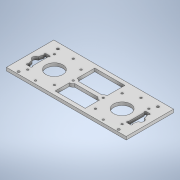
# Autodesk Inventor part: Trunk_lower_waisit_frame
Saved by Autodesk Inventor 2020.4 (Build 244396000, 396)
## iProperties
Created: 2021-09-21
Part Number: Trunk_lower_waisit_frame
Material: アルミニウム 2014-T4
Document SubType Name: Modeling
Designer: Masato Kubotera
Density: 2.8 g/cm^3
Appearance: 滑らか - 淡い灰色
Mass: 76.4309 g
Surface Area: 174.27 cm^2
Volume: 27.2967 cm^3
Description: A2017 T4
Author: Masato Kubotera
Autodesk Inventor part; units mm, degrees
ref_plane "YZ Plane" through (0, 0, 0) normal (1, 0, 0) x (0, 1, 0)
ref_plane "XZ Plane" through (0, 0, 0) normal (0, 1, 0) x (-1, 0, 0)
ref_plane "XY Plane" through (0, 0, 0) normal (0, 0, 1) x (1, 0, 0)
sketch "スケッチ1" plane through (0, 0, 0) normal (0, 0, 1) x (1, 0, 0)
  line L0 (-77.7962, 30.75) -> (77.7962, 30.75)
  line L1 (77.7962, -30.75) -> (-77.7962, -30.75)
  line L2 (-77.7962, 30.75) -> (77.7962, -30.75) construction
  line L3 (77.7962, 30.75) -> (-77.7962, -30.75) construction
  line L4 (0, 30.75) -> (0, -30.75) construction
  circle A0 centre (-44, 2.25) radius 10.5 construction
  line L5 (-57.5, 1.25) -> (-30.5, 1.25) construction
  line L6 (-30.5, 1.25) -> (-30.5, -25.75) construction
  line L7 (-30.5, -25.75) -> (-57.5, -25.75) construction
  line L8 (-57.5, -25.75) -> (-57.5, 1.25) construction
  line L9 (-44, 1.25) -> (-44, -25.75) construction
  line L10 (-57.5, -12.25) -> (-30.5, -12.25) construction
  circle A1 centre (-57.5, 1.25) radius 1.5 construction
  circle A2 centre (-30.5, 1.25) radius 1.5 construction
  line L11 (-67.5, 14.75) -> (-62.5, 14.75) construction
  line L12 (-62.5, 14.75) -> (-62.5, -10.25) construction
  line L13 (-62.5, -10.25) -> (-67.5, -10.25) construction
  line L14 (-67.5, -10.25) -> (-67.5, 14.75) construction
  line L15 (-67.5, 14.75) -> (-62.5, -10.25) construction
  line L16 (-62.5, 14.75) -> (-67.5, -10.25) construction
  line L17 (-67.55, 14.8) -> (-62.45, 14.8)
  line L18 (-62.45, 14.8) -> (-62.45, -10.3)
  line L19 (-62.45, -10.3) -> (-67.55, -10.3)
  line L20 (-67.55, -10.3) -> (-67.55, 14.8)
  line L21 (-67.55, 14.8) -> (-62.45, -10.3) construction
  line L22 (-62.45, 14.8) -> (-67.55, -10.3) construction
  line L23 (-67.55, 2.25) -> (-62.45, 2.25) construction
  line L24 (-65, 14.8) -> (-65, -10.3) construction
  arc A3 (-67.55, 14.8) -> (-67.55, 12.7) centre (-67.55, 13.75) ccw
  arc A4 (-62.45, 12.7) -> (-62.45, 14.8) centre (-62.45, 13.75) ccw
  arc A5 (-67.55, -8.2) -> (-67.55, -10.3) centre (-67.55, -9.25) ccw
  arc A6 (-62.45, -10.3) -> (-62.45, -8.2) centre (-62.45, -9.25) ccw
  circle A7 centre (-65, 27.75) radius 1.55
  line L25 (-10.125, -17.25) -> (-15.125, -17.25) construction
  circle A8 centre (-65, -23.25) radius 1.55
  circle A9 centre (-44, 2.25) radius 11
  line L26 (77.7962, 2.25) -> (-77.7962, 2.25) construction
  line L27 (-60, 14.25) -> (-28, 14.25) construction
  line L28 (-28, 14.25) -> (-28, -28.75) construction
  line L29 (-28, -28.75) -> (-60, -28.75) construction
  line L30 (-60, -28.75) -> (-60, 14.25) construction
  line L31 (-60, 14.25) -> (-28, -28.75) construction
  line L32 (-28, 14.25) -> (-60, -28.75) construction
  line L33 (-77.7962, 30.75) -> (-77.7962, -30.75)
  line L34 (77.7962, 30.75) -> (77.7962, -30.75)
  circle A10 centre (-44, 2.25) radius 12.5 construction
  circle A11 centre (-44, 2.25) radius 20.5 construction
  circle A12 centre (-44, 2.25) radius 28.5 construction
  circle A13 centre (-44, 26.75) radius 1.25
  circle A14 centre (-61.3241, 19.5741) radius 1.25
  circle A15 centre (-68.5, 2.25) radius 1.25
  circle A16 centre (-61.3241, -15.0741) radius 1.25
  circle A17 centre (-44, -22.25) radius 1.25
  circle A18 centre (-26.6759, -15.0741) radius 1.25
  circle A19 centre (-19.5, 2.25) radius 1.25
  circle A20 centre (-26.6759, 19.5741) radius 1.25
  line L35 (-77.7962, -10.0287) -> (-77.7962, -30.75)
  circle A21 centre (57.5, 1.25) radius 1.5 construction
  circle A22 centre (30.5, 1.25) radius 1.5 construction
  line L36 (67.55, 14.8) -> (62.45, 14.8)
  line L37 (62.45, 14.8) -> (62.45, -10.3)
  line L38 (62.45, -10.3) -> (67.55, -10.3)
  line L39 (67.55, -10.3) -> (67.55, 14.8)
  arc A23 (67.55, 12.7) -> (67.55, 14.8) centre (67.55, 13.75) ccw
  arc A24 (62.45, 14.8) -> (62.45, 12.7) centre (62.45, 13.75) ccw
  arc A25 (62.45, -8.2) -> (62.45, -10.3) centre (62.45, -9.25) ccw
  arc A26 (67.55, -10.3) -> (67.55, -8.2) centre (67.55, -9.25) ccw
  circle A27 centre (65, 27.75) radius 1.55
  circle A28 centre (65, -23.25) radius 1.55
  circle A29 centre (44, 2.25) radius 11
  circle A30 centre (44, 26.75) radius 1.25
  circle A31 centre (61.3241, 19.5741) radius 1.25
  circle A32 centre (68.5, 2.25) radius 1.25
  circle A33 centre (61.3241, -15.0741) radius 1.25
  circle A34 centre (44, -22.25) radius 1.25
  circle A35 centre (26.6759, -15.0741) radius 1.25
  circle A36 centre (19.5, 2.25) radius 1.25
  circle A37 centre (26.6759, 19.5741) radius 1.25
  line L40 (77.7962, -10.0287) -> (77.7962, -30.75)
  line L41 (-68.5, 2.25) -> (-73.5, 2.25) construction
  circle A38 centre (-26.6759, -15.0741) radius 6.25 construction
  circle A39 centre (-44, 2.25) radius 24.5 construction
  circle A40 centre (-30.5, -25.75) radius 2.4 construction
  arc A41 (-47.969, 27.2469) -> (-58.8689, 22.732) centre (-44, 2.25) ccw
  arc A42 (-44, 30.75) -> (-47.969, 27.2469) centre (-44, 26.75) ccw
  arc A43 (-58.8689, 22.732) -> (-64.482, 17.1189) centre (-61.3241, 19.5741) ccw
  arc A44 (-64.482, 17.1189) -> (-68.9969, 6.219) centre (-44, 2.25) ccw
  arc A45 (-68.9969, 6.219) -> (-68.9969, -1.719) centre (-68.5, 2.25) ccw
  arc A46 (-68.9969, -1.719) -> (-66.275, -9.7675) centre (-44, 2.25) ccw
  line L42 (-77.7962, -16.309) -> (-77.7962, -10.0287)
  arc A47 (58.8689, 22.732) -> (47.969, 27.2469) centre (44, 2.25) ccw
  arc A48 (47.969, 27.2469) -> (44, 30.75) centre (44, 26.75) ccw
  arc A49 (64.482, 17.1189) -> (58.8689, 22.732) centre (61.3241, 19.5741) ccw
  arc A50 (68.9969, 6.219) -> (64.482, 17.1189) centre (44, 2.25) ccw
  arc A51 (68.9969, -1.719) -> (68.9969, 6.219) centre (68.5, 2.25) ccw
  arc A52 (66.275, -9.7675) -> (68.9969, -1.719) centre (44, 2.25) ccw
  line L43 (77.7962, -16.309) -> (77.7962, -10.0287)
  line L44 (19.5, 25.75) -> (-19.5, 25.75)
  line L45 (-19.5, 25.75) -> (-19.5, 7.25)
  circle A53 centre (-65, 27.75) radius 2.75 construction
  line L46 (-15.1699, 4.75) -> (15.1699, 4.75)
  arc A54 (-15.1699, 4.75) -> (-19.5, 7.25) centre (-19.5, 2.25) ccw
  line L47 (19.5, 25.75) -> (19.5, 7.25)
  arc A55 (19.5, 7.25) -> (15.1699, 4.75) centre (19.5, 2.25) ccw
  line L48 (-15.1699, -0.25) -> (15.1699, -0.25)
  arc A56 (-19.5, -2.75) -> (-15.1699, -0.25) centre (-19.5, 2.25) ccw
  arc A57 (15.1699, -0.25) -> (19.5, -2.75) centre (19.5, 2.25) ccw
  line L49 (-19.5, -2.75) -> (-19.5, -25.75)
  line L50 (-19.5, -25.75) -> (19.5, -25.75)
  line L51 (19.5, -25.75) -> (19.5, -2.75)
  point P0 (0, 0)
  point P1 (-65, 2.25)
  point P2 (-62.45, 12.7)
  point P3 (-62.45, -8.2)
  point P4 (-67.55, -8.2)
  point P5 (-44, -7.25)
  point P6 (62.45, -8.2)
  point P7 (62.45, 12.7)
  point P8 (27.9147, 19.7411)
  point P9 (27.51, 18.6431)
  point P10 (-27.51, 18.6431)
  point P11 (-27.9147, 19.7411)
  point P12 (-26.4271, 21.76)
  point P13 (-26.9247, 21.76)
  point P14 (-27.51, 20.5051)
  point P15 (27.51, 20.5051)
  point P16 (26.9247, 21.76)
  point P17 (26.4271, 21.76)
  point P18 (-47, 30.75)
  point P19 (47, 30.75)
  point P20 (-65, 2.25)
  point P21 (-67.0074, 12.7979)
  point P22 (-67.45, 11.7733)
  point P23 (-67.45, 2.9282)
  point P24 (-67.45, 1.5718)
  point P25 (-67.45, -7.2733)
  point P26 (-67.0074, -8.2979)
  point P27 (67.0074, -8.2979)
  point P28 (67.45, -7.2733)
  point P29 (67.45, 1.5718)
  point P30 (67.45, 2.9282)
  point P31 (67.45, 11.7733)
  point P32 (67.0074, 12.7979)
  point P33 (-67.55, 11.5233)
  point P34 (-65.9794, 14.8)
  point P35 (-67.55, 3.0624)
  point P36 (-67.55, 1.4376)
  point P37 (-67.55, -7.0233)
  point P38 (65.9794, 14.8)
  point P39 (67.55, 11.5233)
  point P40 (67.55, 1.4376)
  point P41 (67.55, 3.0624)
  point P42 (67.55, -7.0233)
  dimension "d3" = 21
  dimension "d4" = 27
  dimension "d5" = 3
  dimension "d7" = 27
  dimension "d8" = 5
  dimension "d9" = 25
  dimension "d10" = 0.05
  dimension "d11" = 0.05
  dimension "d12" = 1.05
  dimension "d13" = 3.1
  dimension "d19" = 3.1
  dimension "d21" = 6
  dimension "d24" = 3
  dimension "d29" = 0.5
  dimension "d34" = 11.5
  dimension "d45" = 32
  dimension "d46" = 43
  dimension "d47" = 9.5
  dimension "d71" = 44
  dimension "d73" = 1
  dimension "d78" = 28.5
  dimension "d79" = 33
  dimension "d80" = 25
  dimension "d81" = 41
  dimension "d82" = 8
  dimension "d84" = 2.5
  dimension "d85" = 24.5
  dimension "d88" = 360
  dimension "d90" = 2
  dimension "d93" = 4
  dimension "d94" = 5
  dimension "d97" = 5
  dimension "d101" = 4.8
  dimension "d105" = 4
  dimension "d106" = 25.31
  dimension "d107" = 4
  dimension "d108" = 25.31
  dimension "d109" = 25.31
  dimension "d110" = 4
  dimension "d113" = 5.5
  dimension "d114" = 5
  dimension "d117" = 5
  dimension "d118" = 5
  dimension "d122" = 5
  dimension "d123" = 16
  dimension "d124" = 13
  dimension "d125" = 67.5
  constraints: 104 end point, 58 centre point, 56 symmetric about line, 50 point on circle, 19 midpoint, 17 coincident, 16 point on line, 10 parallel, 9 perpendicular, 8 horizontal, 4 vertical, 47 other
  measures "d3" diameter of A0
  measures "d4" distance of L6.end L7.end
  measures "d5" diameter of A1
  measures "d7" distance of L6.end L5.end
  measures "d8" distance of L12.end L13.end
  measures "d9" distance of L11.end L12.end
  measures "d10" distance between parallel lines of L17 L11
  measures "d11" distance between parallel lines of L18 L12
  measures "d12" radius of A3
  measures "d13" diameter of A7
  measures "d19" diameter of A8
  measures "d21" vertical distance of L25.start A8.centre
  measures "d24" vertical distance of L4.start A7.centre
  measures "d29" radial gap between concentric circles of A0 A9
  measures "d34" distance from line of A2.centre L13
  measures "d45" distance of L28.end L29.end
  measures "d46" distance of L27.end L28.end
  measures "d47" distance of point (-44, -7.25) A9.centre
  measures "d71" horizontal distance of point (0, 0) A0.centre
  measures "d73" distance of L9.start A9.centre
  measures "d78" distance from line of L26.end L0
  measures "d79" distance from line of L1 L26.end
  measures "d80" diameter of A10
  measures "d81" diameter of A11
  measures "d82" radial gap between concentric circles of A12 A11
  measures "d84" diameter of A13
  measures "d85" distance of A0.centre A13.centre
  measures "d90" vertical distance of L1.end L29.end
  measures "d93" distance from line of A13.centre L0
  measures "d94" distance of L41.start L41.end
  measures "d97" radial gap between concentric circles of A18 A38
  measures "d101" diameter of A40
  measures "d105" radius of A42
  measures "d106" radius of A41
  measures "d107" radius of A43
  measures "d108" radius of A44
  measures "d109" radius of A46
  measures "d110" radius of A45
  measures "d113" diameter of A53
  measures "d114" distance from line of L44.end L0
  measures "d117" distance between parallel lines of L48 L46
  measures "d118" distance between parallel lines of L1 L50
  measures "d122" radius of A54
  measures "d123" distance from line of L11.end L0
  measures "d124" distance from line of A8.centre L13
  measures "d125" distance between parallel lines of L14 L4
extrude "押し出し1" add sketch "スケッチ1" along normal blind 4
equation "\"d11\" = d10"
